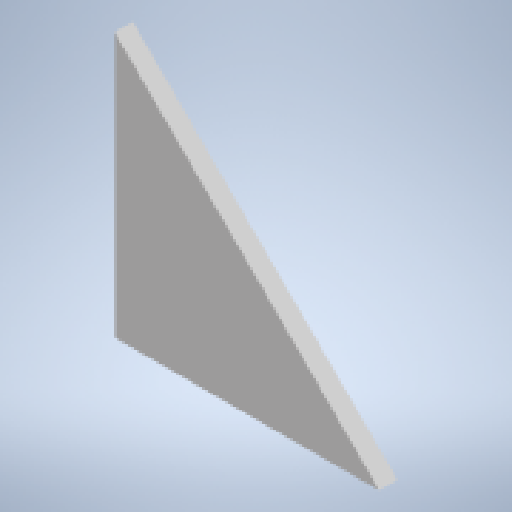
# Autodesk Inventor part: 145x145(li)
Saved by Autodesk Inventor 2023 (Build 270158000, 158)
## iProperties
Created: 2025-04-11
Part Number: 145x145(li)
Material: Generic
Document SubType Name: Modeling
Designer: huyqu
Density: 1 g/cm^3
Appearance: Default
Author: huyqu
Autodesk Inventor part; units mm, degrees
ref_plane "YZ Plane" through (0, 0, 0) normal (1, 0, 0) x (0, 1, 0)
ref_plane "XZ Plane" through (0, 0, 0) normal (0, 1, 0) x (-1, 0, 0)
ref_plane "XY Plane" through (0, 0, 0) normal (0, 0, 1) x (1, 0, 0)
sketch "Sketch1" plane through (0, 0, 0) normal (0, 0, 1) x (1, 0, 0)
  line L0 (0, 0) -> (0, 145)
  line L1 (0, 145) -> (145, 0)
  line L2 (145, 0) -> (0, 0)
  dimension "d0" = 145
  dimension "d1" = 145
  constraints: 6 end point, 1 perpendicular, 1 vertical
  measures "d0" distance of L0.start L0.end
  measures "d1" distance of L1.end L0.start
extrude "Extrusion1" add sketch "Sketch1" along normal blind 10
sketch "Sketch2" plane through (0, 0, 0) normal (0, -1, 0) x (1, 0, 0)
  line L0 (145, 0) -> (145, 10) projected
  line L1 (145, 5) -> (0, 5)
  circle A0 centre (105, 5) radius 3
  circle A1 centre (40, 5) radius 3
  line L2 (0, 0) -> (0, 10) projected
  dimension "d4" = 6
  dimension "d5" = 6
  dimension "d6" = 40
  dimension "d7" = 40
  constraints: 2 centre point, 2 end point, 2 point on line, 1 horizontal, 1 midpoint
  measures "d4" diameter of A0
  measures "d5" diameter of A1
  measures "d6" distance from line of A0.centre L0
  measures "d7" distance from line of L2 A1.centre
hole "Hole1" at (105, 0, 5) at (40, 0, 5) direction (0, 1, 0) diameter 4.917 depth 17.1 thread size "M6x1" class "6H" standard "ISO Metric profile"
sketch "Sketch3" plane through (0, 0, 0) normal (-1, 0, 0) x (0, 0, 1)
  line L0 (0, 145) -> (10, 145) projected
  line L1 (5, 145) -> (5, 0)
  line L2 (0, 0) -> (10, 0) projected
  circle A0 centre (5, 105) radius 3
  circle A1 centre (5, 40) radius 3
  dimension "d15" = 6
  dimension "d16" = 6
  dimension "d17" = 40
  dimension "d18" = 40
  constraints: 2 centre point, 2 end point, 2 midpoint, 2 point on line
  measures "d15" diameter of A0
  measures "d16" diameter of A1
  measures "d17" distance from line of A0.centre L0
  measures "d18" distance from line of L2 A1.centre
hole "Hole2" at (0, 105, 5) at (0, 40, 5) direction (1, 0, 0) diameter 5.1881 depth 17.1 thread size "M6x0.75" class "6H" standard "ISO Metric profile"
sketch "Sketch4" plane through (0, 0, 0) normal (-1, 0, 0) x (0, 0, 1)
  point P0 (0, 0)
body "Solid1"
